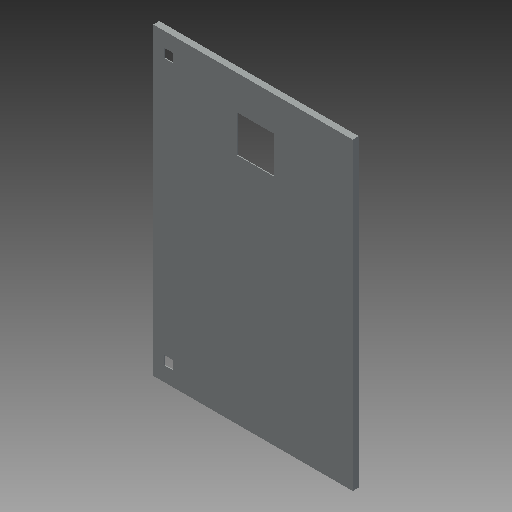
# Autodesk Inventor part: 1130_01_03 (2)
Saved by Autodesk Inventor 2019.3 (Build 233278000, 278)
## iProperties
Category: PARTsolutions
Company: RITTAL
Created: 2018-11-14
Part Number: 1130_01_03 (2)
Material: Generic
Catalog Web Link: www.cadenas.de
Description: Tür rechts AE-Tür rechts AE
Vendor: RITTAL
Document SubType Name: Modeling
Designer: psadmin
Manufacturer: RITTAL
Mass: 943.347 g
Surface Area: 8381.49 cm^2
Volume: 943.347 cm^3
Density: 1 g/cm^3
Appearance: PSOLRGB-195-201-196
PSOL_IDENT_0: {$CADENAS_DATA\23d-libs\rittal_usa\schaltschranksys\kompakt_schaltschr\ae\parts_ae\tuer_rechts_ae.pr
PSOL_IDENT_1: j},201 {VTYP=3D},{NB=1130_01_03 (2)},{LINA=1130_01_03 (2)},{NN=Tür rechts AE},{DATE=08.11.2018 06:46
PSOL_IDENT_2: :30},{GEOMDATE=07.07.2014 12:39:29},{VERSION=v140715130753},{LINEID=220},{WBVAR=DETAIL},{WBNUMERIC=D
PSOL_IDENT_3: ETAIL}  {NB=1130_01_03 (2)},{LINA=1130_01_03 (2)},{KT=DUMMY},{BEST=1130},{VERS=1},{DETAIL=2},{BEZ1=M
PSOL_IDENT_4: IN},{BEZ2=MIN},{BEZ3=MIN},{A=1000.000},{B=760.000},{C=300.000},{D=303.000},{E=113.000},{F=70.000},{G=
PSOL_IDENT_5: 30.000},{H=705.000},{I=667.200},{J=2.000},{K=730.000},{P=905.000},{Q=944.000},{R=495.000},{S=755.000
PSOL_IDENT_6: },{T=616.400},{U=675.000},{UU=575.000},{V=27.000},{VV=23.000},{W=698.000},{WW=598.000},{X=424.000},{
PSOL_IDENT_7: Y=436.000},{B1=1000},{H1=760},{T1=300},{F1=944},{G1=730},{S1=3.0},{GEW=56.0},{XX=1.800}
NN: Tür rechts AE
NT: Tür rechts AE
NB: 1130_01_03 (2)
NBSYN: $BEST._01_03 ($DETAIL.)
LINA: 1130_01_03 (2)
BEST: 1130
VERS: 1
DETAIL: 2
BEZ1: 0
BEZ2: 0
BEZ3: 0
A: 1000
B: 760
C: 300
D: 303
E: 113
F: 70
G: 30
H: 705
I: 667.2
J: 2
K: 730
P: 905
Q: 944
R: 495
S: 755
T: 616.4
U: 675
UU: 575
V: 27
VV: 23
W: 698
WW: 598
X: 424
Y: 436
B1: 1000
H1: 760
T1: 300
F1: 944
G1: 730
S1: 3
GEW: 56
XX: 1.8
SUPPLIER: RITTAL
ARTICLENO: 1130_01_03 (2)
BOMINFO: 1130_01_03 (2)
CREATOR: CADENAS GmbH
Title: 1130_01_03 (2)
Author: Cadenas PARTsolutions
Comments: Tür rechts AE
Autodesk Inventor part; units mm, degrees
sketch "Skizze_1" plane through (0, 0, 0) normal (0, 0, 1) x (1, 0, 0)
  line L0 (-247.5, 377.5) -> (-247.5, -377.5)
  line L1 (-247.5, -377.5) -> (247.5, -377.5)
  line L2 (247.5, -377.5) -> (247.5, 377.5)
  line L3 (247.5, 377.5) -> (-247.5, 377.5)
  constraints: 8 end point
extrude "Extrusion1" add sketch "Skizze_1" against normal blind 15
sketch "Skizze_2" plane through (0, 0, 0) normal (1, 0, 0) x (0, 0, -1)
  line L0 (2, 375.5) -> (2, -375.5)
  line L1 (2, -375.5) -> (17, -375.5)
  line L2 (17, -375.5) -> (17, 375.5)
  line L3 (17, 375.5) -> (2, 375.5)
  constraints: 8 end point
extrude "Extrusion2" cut sketch "Skizze_2" along normal mid plane 491
sketch "Skizze_3" plane through (0, 0, -2) normal (0, 0, 1) x (1, 0, 0)
  line L0 (-245.5, 361.5) -> (231.5, 361.5)
  line L1 (231.5, 361.5) -> (231.5, -361.5)
  line L2 (231.5, -361.5) -> (-245.5, -361.5)
  line L3 (-245.5, -361.5) -> (-245.5, -373.5)
  line L4 (-245.5, -373.5) -> (243.5, -373.5)
  line L5 (243.5, -373.5) -> (243.5, 373.5)
  line L6 (243.5, 373.5) -> (-245.5, 373.5)
  line L7 (-245.5, 373.5) -> (-245.5, 361.5)
  constraints: 16 end point
sketch "Skizze_21" plane through (0, -320.6, 0) normal (0, 1, 0) x (1, 0, 0)
  arc A0 (241.2, 12.35) -> (241.2, 4.05) centre (241.2, 8.2) ccw
  line L0 (241.2, 4.05) -> (245.5, 4.05)
  line L1 (245.5, 4.05) -> (245.5, 5.5)
  line L2 (245.5, 5.5) -> (241.2, 5.5)
  arc A1 (241.2, 10.9) -> (241.2, 5.5) centre (241.2, 8.2) ccw
  line L3 (241.2, 10.9) -> (245.5, 10.9)
  line L4 (245.5, 10.9) -> (245.5, 12.35)
  line L5 (245.5, 12.35) -> (241.2, 12.35)
  constraints: 12 end point, 4 point on circle, 2 centre point
extrude "Extrusion3" add sketch "Skizze_21" along normal mid plane 26
sketch "Skizze_22" plane through (0, 320.6, 0) normal (0, 1, 0) x (1, 0, 0)
  arc A0 (241.2, 12.35) -> (241.2, 4.05) centre (241.2, 8.2) ccw
  line L0 (241.2, 4.05) -> (245.5, 4.05)
  line L1 (245.5, 4.05) -> (245.5, 5.5)
  line L2 (245.5, 5.5) -> (241.2, 5.5)
  arc A1 (241.2, 10.9) -> (241.2, 5.5) centre (241.2, 8.2) ccw
  line L3 (241.2, 10.9) -> (245.5, 10.9)
  line L4 (245.5, 10.9) -> (245.5, 12.35)
  line L5 (245.5, 12.35) -> (241.2, 12.35)
  constraints: 12 end point, 4 point on circle, 2 centre point
extrude "Extrusion4" add sketch "Skizze_22" along normal mid plane 26
sketch "Skizze_24" plane through (0, 0, 0) normal (0, 0, 1) x (1, 0, 0)
  line L0 (-221.05, -318.95) -> (-221.05, -341.05)
  line L1 (-221.05, -341.05) -> (-198.95, -341.05)
  line L2 (-198.95, -341.05) -> (-198.95, -318.95)
  line L3 (-198.95, -318.95) -> (-221.05, -318.95)
  constraints: 8 end point
extrude "Extrusion5" cut sketch "Skizze_24" against normal blind 2
sketch "Skizze_41" plane through (0, 0, 0) normal (0, 0, 1) x (1, 0, 0)
  line L0 (-221.05, 341.05) -> (-221.05, 318.95)
  line L1 (-221.05, 318.95) -> (-198.95, 318.95)
  line L2 (-198.95, 318.95) -> (-198.95, 341.05)
  line L3 (-198.95, 341.05) -> (-221.05, 341.05)
  constraints: 8 end point
extrude "Extrusion6" cut sketch "Skizze_41" against normal blind 2
sketch "Skizze_23" plane through (-247.5, 0, 0) normal (1, 0, 0) x (0, 0, -1)
  arc A0 (13.25, 372.2142) -> (13.25, 354.7858) centre (15.5, 363.5) ccw
  arc A1 (15.5, 351.881) -> (13.25, 354.7858) centre (12.5, 351.881) ccw
  line L0 (15.5, 351.881) -> (15.5, 375.119)
  arc A2 (13.25, 372.2142) -> (15.5, 375.119) centre (12.5, 375.119) ccw
  constraints: 6 point on circle, 3 centre point, 2 end point
extrude "Extrusion7" cut sketch "Skizze_23" along normal blind 3
sketch "Skizze_26" plane through (-247.5, 0, 0) normal (1, 0, 0) x (0, 0, -1)
  arc A0 (13.25, -354.7858) -> (13.25, -372.2142) centre (15.5, -363.5) ccw
  arc A1 (15.5, -375.119) -> (13.25, -372.2142) centre (12.5, -375.119) ccw
  line L0 (15.5, -375.119) -> (15.5, -351.881)
  arc A2 (13.25, -354.7858) -> (15.5, -351.881) centre (12.5, -351.881) ccw
  constraints: 6 point on circle, 3 centre point, 2 end point
extrude "Extrusion8" cut sketch "Skizze_26" along normal blind 3
extrude "Extrusion9" add sketch "Skizze_3" against normal blind 6.5
ref_plane "tuer_XY" through (241.2, -320.6, -8.2) normal (0, 1, 0) x (1, 0, 0)
ref_plane "tuer_YZ" through (241.2, -320.6, -8.2) normal (1, 0, 0) x (0, 0, -1)
ref_plane "tuer_ZX" through (241.2, -320.6, -8.2) normal (0, 0, -1) x (0, 1, 0)
ref_plane "verschluss_XY" through (-210, -330, 0) normal (0, 0, 1) x (1, 0, 0)
ref_plane "verschluss_YZ" through (-210, -330, 0) normal (1, 0, 0) x (0, 1, 0)
ref_plane "verschluss_ZX" through (-210, -330, 0) normal (0, 1, 0) x (0, 0, 1)
ref_plane "verschluss2_XY" through (-210, 330, 0) normal (0, 0, 1) x (1, 0, 0)
ref_plane "verschluss2_YZ" through (-210, 330, 0) normal (1, 0, 0) x (0, 1, 0)
ref_plane "verschluss2_ZX" through (-210, 330, 0) normal (0, 1, 0) x (0, 0, 1)
sketch "Эскиз10" plane through (0, 0, 0) normal (0, 0, 1) x (1, 0, 0)
  line L0 (-39.5, 292.5) -> (52.5, 292.5)
  line L1 (52.5, 292.5) -> (52.5, 200.5)
  line L2 (52.5, 200.5) -> (-39.5, 200.5)
  line L3 (-39.5, 200.5) -> (-39.5, 292.5)
  line L4 (247.5, -377.5) -> (247.5, 377.5) projected
  line L5 (247.5, 377.5) -> (-247.5, 377.5) projected
  point P0 (0, 0)
  dimension "d20" = 92
  dimension "d21" = 92
  dimension "d22" = 195
  dimension "d23" = 85
  constraints: 8 end point, 2 parallel, 1 horizontal, 1 perpendicular
  measures "d20" distance of L1.end L2.end
  measures "d21" distance of L0.end L1.end
  measures "d22" distance between parallel lines of L4 L1
  measures "d23" distance between parallel lines of L5 L0
extrude "Выдавливание10" cut sketch "Эскиз10" against normal blind 10
body "Solid1"
